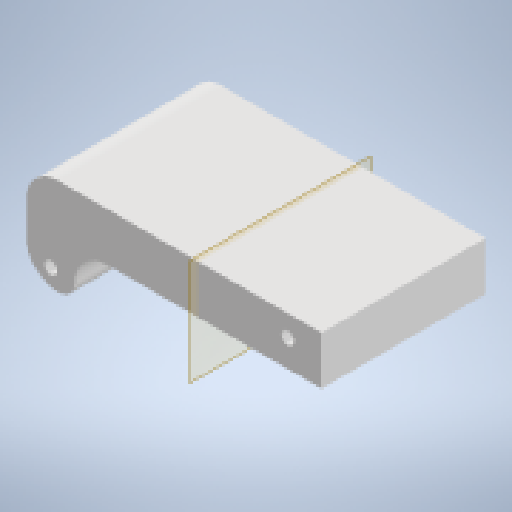
# Autodesk Inventor part: Фиксатор головы
Saved by Autodesk Inventor 2023.2 (Build 272271030, 271C)
## iProperties
Created: 2024-02-24
Part Number: Фиксатор головы
Material: Типовые
Document SubType Name: Modeling
Designer: I9232
Density: 1 g/cm^3
Appearance: По умолчанию
Author: I9232
Autodesk Inventor part; units mm, degrees
ref_plane "XZ Plane" through (0, 0, 0) normal (0, 1, 0) x (-1, 0, 0)
ref_plane "XY Plane" through (0, 0, 0) normal (0, 0, 1) x (1, 0, 0)
sketch "Эскиз1" plane through (0, 0, 0) normal (0, 0, 1) x (1, 0, 0)
  line L0 (-32.5, -7.5) -> (32.5, -7.5)
  line L1 (32.5, -7.5) -> (32.5, 7.5)
  line L2 (32.5, 7.5) -> (-32.5, 7.5)
  line L3 (-32.5, -7.5) -> (32.5, 7.5) construction
  line L4 (32.5, -7.5) -> (-32.5, 7.5) construction
  line L5 (-32.5, 7.5) -> (-47.5, 7.5)
  line L6 (-47.5, 7.5) -> (-47.5, -22.5)
  line L7 (-47.5, -22.5) -> (-32.5, -22.5)
  line L8 (-32.5, -22.5) -> (-32.5, -7.5)
  line L9 (-32.5, -7.5) -> (-32.5, 7.5)
  point P0 (0, 0)
  dimension "d5" = 65
  dimension "d6" = 15
  dimension "d7" = 30
  dimension "d8" = 15
  constraints: 20 end point, 3 parallel, 3 perpendicular, 2 horizontal, 2 midpoint
  measures "d5" distance of L1.end L2.end
  measures "d6" distance of L2.end L5.end
  measures "d7" distance of L5.end L6.end
  measures "d8" distance of L0.end L1.end
extrude "Выдавливание1" add sketch "Эскиз1" along normal mid plane 57
sketch "Эскиз2" plane through (0, 0, 28.5) normal (0, 0, 1) x (1, 0, 0)
  circle A0 centre (-40, -17) radius 2
  circle A1 centre (27.758, 0.9216) radius 2
  line L0 (-47.5, -22.5) -> (-32.5, -22.5) projected
  line L1 (-40, -22.5) -> (-40, 7.5) construction
  line L2 (32.5, 7.5) -> (-47.5, 7.5) projected
  line L3 (32.5, -7.5) -> (32.5, 7.5) projected
  circle A2 centre (27.758, 0.9216) radius 2
  point P0 (0, 0)
  dimension "d9" = 4
  dimension "d10" = 5.5
  constraints: 3 centre point, 2 end point, 2 point on line, 1 coincident, 1 equal radius, 1 midpoint, 1 vertical
  measures "d9" diameter of A0
  measures "d10" distance from line of L0 A0.centre
extrude "Выдавливание2" cut sketch "Эскиз2" against normal up to surface (57 mm away)
fillet "Сопряжение1" radius 10 3 edges at (-47.5, 7.5, 0) (-47.5, -22.5, 0) (-32.5, -7.5, 0)
fillet "Сопряжение2" radius 5 1 edges at (-32.5, -22.5, 0)
